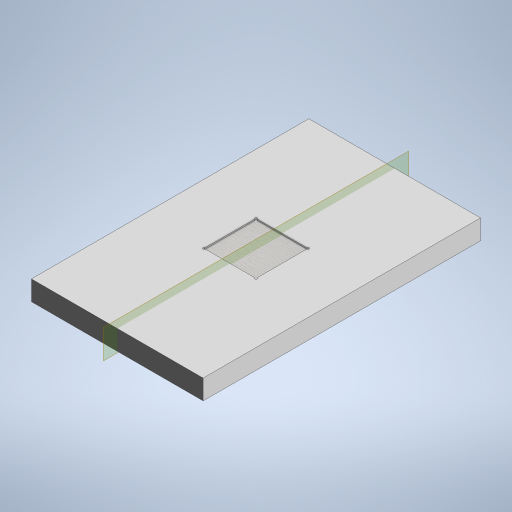
# Autodesk Inventor part: Monitor
Saved by Autodesk Inventor 2023 (Build 270158000, 158)
## iProperties
Created: 2023-02-09
Part Number: Monitor
Material: Generic
Document SubType Name: Modeling
Designer: rosam
Density: 1 g/cm^3
Appearance: Default
Author: rosam
Autodesk Inventor part; units mm, degrees
ref_plane "YZ Plane" through (0, 0, 0) normal (1, 0, 0) x (0, 1, 0)
ref_plane "XZ Plane" through (0, 0, 0) normal (0, 1, 0) x (-1, 0, 0)
ref_plane "XY Plane" through (0, 0, 0) normal (0, 0, 1) x (1, 0, 0)
sketch "Sketch1" plane through (0, 0, 0) normal (0, 1, 0) x (-1, 0, 0)
  line L0 (165.1, 266.7) -> (-165.1, 266.7)
  line L1 (-165.1, 266.7) -> (-165.1, -266.7)
  line L2 (-165.1, -266.7) -> (165.1, -266.7)
  line L3 (165.1, -266.7) -> (165.1, 266.7)
  point P0 (0, 0)
  dimension "d0" = 533.4
  dimension "d1" = 330.2
  dimension "d2" = 266.7
  dimension "d3" = 165.1
  constraints: 8 end point, 2 parallel, 1 horizontal, 1 perpendicular
  measures "d0" distance of L2.end L0.start
  measures "d1" distance of L0.start L0.end
  measures "d2" distance from line of point (0, 0) L0
  measures "d3" distance from line of point (0, 0) L3
extrude "Extrusion1" add sketch "Sketch1" along normal blind 38.1
sketch "Sketch2" plane through (0, 38.1, 0) normal (0, 1, 0) x (1, 0, 0)
  line L0 (-165.1, -266.7) -> (165.1, -266.7) projected
  line L1 (165.1, 266.7) -> (-165.1, 266.7) projected
  line L2 (-50.038, -50.038) -> (50.038, -50.038)
  line L3 (50.038, -50.038) -> (50.038, 50.038)
  line L4 (50.038, 50.038) -> (-50.038, 50.038)
  line L5 (-50.038, 50.038) -> (-50.038, -50.038)
  circle A0 centre (-50.038, 50.038) radius 2.0003
  circle A1 centre (50.038, 50.038) radius 2.0003
  circle A2 centre (50.038, -50.038) radius 2.0003
  circle A3 centre (-50.038, -50.038) radius 2.0003
  point P0 (-50.038, -48.0378)
  point P1 (-48.0377, -50.038)
  point P2 (48.0378, -50.038)
  point P3 (50.038, -48.0378)
  point P4 (50.038, 48.0378)
  point P5 (48.0378, 50.038)
  point P6 (-48.0377, 50.038)
  point P7 (-50.038, 48.0378)
  dimension "d20" = 100.076
  dimension "d21" = 100.076
  dimension "d22" = 115.062
  dimension "d23" = 115.062
  dimension "d24" = 216.662
  dimension "d25" = 216.662
  dimension "d26" = 4.0005
  dimension "d27" = 4.0005
  dimension "d28" = 4.0005
  dimension "d29" = 4.0005
  constraints: 8 end point, 4 centre point, 4 coincident, 2 parallel, 1 horizontal, 1 perpendicular
  measures "d20" distance of L4.end L2.start
  measures "d21" distance of L2.start L2.end
  measures "d22" horizontal distance of L0.start L2.start
  measures "d23" horizontal distance of L0.end L2.end
  measures "d24" distance from line of L1 L3.end
  measures "d25" vertical distance of L0.end L2.end
  measures "d26" diameter of A0
  measures "d27" diameter of A1
  measures "d28" diameter of A2
  measures "d29" diameter of A3
extrude "Extrusion2" cut sketch "Sketch2" against normal blind 2.54
ref_plane "Work Plane1" through (0, 0, -266.7) normal (-1, 0, 0) x (0, 0, 1)
equation "\"d2\" = 0.5 * d0"
equation "\"d3\" = 0.5 * d1"
equation "\"d22\" = d23"
equation "\"d24\" = d25"
equation "\"d26\" = d29"
equation "\"d27\" = d29"
equation "\"d28\" = d29"
body "Solid1"
